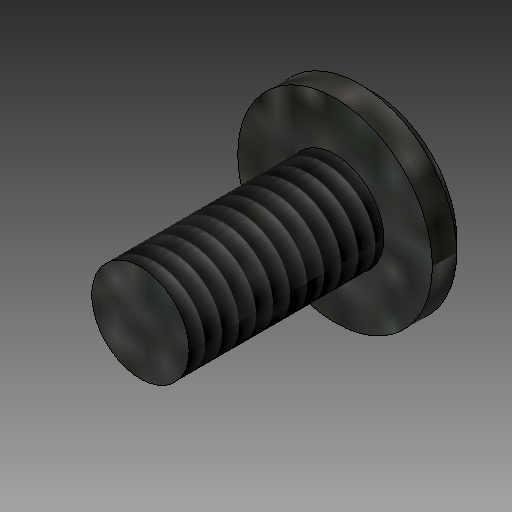
# Autodesk Inventor part: 低頭ねじM4×8
Saved by Autodesk Inventor 2019 (Build 230136000, 136)
## iProperties
Created: 2019-11-28
Part Number: 低頭ねじM4×8
Material: 鋼
Document SubType Name: Modeling
Designer: tanjihayato
Density: 7.85 g/cm^3
Appearance: プレート
Mass: 1.31662 g
Surface Area: 2.41467 cm^2
Volume: 0.167722 cm^3
Author: tanjihayato
Autodesk Inventor part; units mm, degrees
ref_plane "YZ Plane" through (0, 0, 0) normal (1, 0, 0) x (0, 1, 0)
ref_plane "XZ Plane" through (0, 0, 0) normal (0, 1, 0) x (-1, 0, 0)
ref_plane "XY Plane" through (0, 0, 0) normal (0, 0, 1) x (1, 0, 0)
sketch "スケッチ1" plane through (0, 0, 0) normal (0, 0, 1) x (1, 0, 0)
  circle A0 centre (0, 0) radius 4
  circle A1 centre (0, 0) radius 2
  dimension "d0" = 8
  dimension "d1" = 4
  constraints: 2 centre point, 2 coincident
  measures "d0" diameter of A0
  measures "d1" diameter of A1
extrude "押し出し1" add sketch "スケッチ1" against normal blind 1.5 contours A0 | A1
extrude "押し出し2" add sketch "スケッチ1" along normal blind 8 contours A1
sketch "スケッチ2" plane through (0, 0, -1.5) normal (0, 0, -1) x (-1, 0, 0)
  line L0 (-0.5774, 1) -> (0.5774, 1)
  line L1 (0.5774, 1) -> (1.1547, 0)
  line L2 (1.1547, 0) -> (0.5774, -1)
  line L3 (0.5774, -1) -> (-0.5774, -1)
  line L4 (-0.5774, -1) -> (-1.1547, 0)
  line L5 (-1.1547, 0) -> (-0.5774, 1)
  point P0 (0, 0)
  point P1 (0, 0)
  dimension "d6" = 2
  constraints: 12 end point, 1 coincident, 1 horizontal, 13 other
  measures "d6" distance between parallel lines of L3 L0
extrude "押し出し3" cut sketch "スケッチ2" against normal blind 1.5
chamfer "面取り1" distance 0.5 angle 45 1 edges at (-4, 0, -1.5)
thread "ねじ1" size "M4x0.7" class "6g" standard "ANSI Metric M Profile" full length
